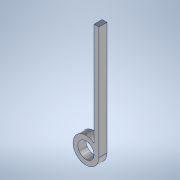
# Autodesk Inventor part: Feder_V1
Saved by Autodesk Inventor 2022 (Build 260153000, 153)
## iProperties
Created: 2022-04-11
Part Number: Feder_V1
Material: Generic
Document SubType Name: Modeling
Designer: richa
Density: 1 g/cm^3
Appearance: Aluminum - Flat
Author: richa
Autodesk Inventor part; units mm, degrees
ref_plane "YZ Plane" through (0, 0, 0) normal (1, 0, 0) x (0, 1, 0)
ref_plane "XZ Plane" through (0, 0, 0) normal (0, 1, 0) x (-1, 0, 0)
ref_plane "XY Plane" through (0, 0, 0) normal (0, 0, 1) x (1, 0, 0)
sketch "Sketch1" plane through (0, 0, 0) normal (0, 0, 1) x (1, 0, 0)
  circle A0 centre (0, 0) radius 5
  circle A1 centre (0, 0) radius 8
  dimension "d0" = 10
  dimension "d1" = 16
  constraints: 2 centre point, 2 coincident
  measures "d0" diameter of A0
  measures "d1" diameter of A1
extrude "Extrusion1" add sketch "Sketch1" along normal blind 5
sketch "Sketch2" plane through (0, 0, 5) normal (0, 0, 1) x (1, 0, 0)
  circle A0 centre (0, 0) radius 8 projected
  line L0 (8, 0) -> (5, 0)
  line L1 (8, 70) -> (8, 0)
  circle A1 centre (0, 0) radius 5 projected
  line L2 (5, 70) -> (5, 0)
  line L3 (5, 70) -> (8, 70)
  point P0 (5, 6.245)
  point P1 (7, 3.873)
  dimension "d4" = 0
  dimension "d9" = 70
  dimension "d11" = 3
  constraints: 8 end point, 2 horizontal, 2 point on circle, 1 parallel, 1 perpendicular, 2 other
  measures "d4" distance from line of point (0, 0) L0
  measures "d9" distance of L1.start L0.start
  measures "d11" distance of L2.start L1.start
extrude "Extrusion2" add sketch "Sketch2" against normal blind 5 contours A0 L2 L3 L1
body "Solid1"
